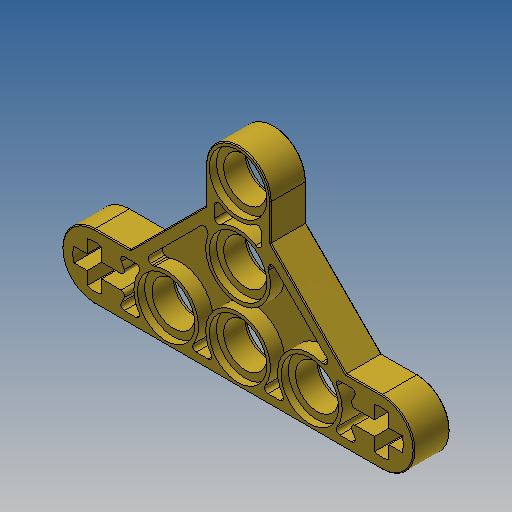
# Autodesk Inventor part: 99773-LtBluishGray
Saved by Autodesk Inventor 2025 (Build 290162010, 162A)
## iProperties
Created: 2014-08-22
Part Number: 99773-LtBluishGray
Material: ABS Plastic
Document SubType Name: Modeling
Designer: D. Kohfeld
Density: 1.06 g/cm^3
Appearance: Yellow
Mass: 0.939287 g
Surface Area: 19.226 cm^2
Volume: 0.88612 cm^3
Author: D. Kohfeld
Autodesk Inventor part; units mm, degrees
ref_plane "YZ Plane" through (0, 0, 0) normal (1, 0, 0) x (0, 1, 0)
ref_plane "XZ Plane" through (0, 0, 0) normal (0, 1, 0) x (-1, 0, 0)
ref_plane "XY Plane" through (0, 0, 0) normal (0, 0, 1) x (1, 0, 0)
sketch "Sketch1" plane through (0, 0, 0) normal (0, 0, 1) x (1, 0, 0)
  circle A0 centre (0, 0) radius 2.4
  circle A1 centre (-8, 0) radius 2.4
  circle A2 centre (-16, 0) radius 2.4 construction
  circle A3 centre (8, 0) radius 2.4
  circle A4 centre (16, 0) radius 2.4 construction
  circle A5 centre (0, 8) radius 2.4
  circle A6 centre (0, 16) radius 2.4
  line L0 (-16, 0) -> (-8, 0) construction
  line L1 (-8, 0) -> (0, 0) construction
  line L2 (0, 0) -> (8, 0) construction
  line L3 (8, 0) -> (16, 0) construction
  line L4 (0, 0) -> (0, 8) construction
  line L5 (0, 8) -> (0, 16) construction
  circle A7 centre (-8, 0) radius 3.6 construction
  circle A8 centre (0, 0) radius 3.6 construction
  circle A9 centre (8, 0) radius 3.6 construction
  circle A10 centre (0, 8) radius 3.6 construction
  circle A11 centre (0, 16) radius 3.6 construction
  line L6 (-3.6, 16) -> (-3.6, 12)
  line L7 (-3.6, 12) -> (-12, 3.6)
  line L8 (-12, 3.6) -> (-16, 3.6)
  arc A12 (-16, 3.6) -> (-16, -3.6) centre (-16, 0) ccw
  line L9 (-16, -3.6) -> (16, -3.6)
  arc A13 (16, -3.6) -> (16, 3.6) centre (16, 0) ccw
  line L10 (16, 3.6) -> (12, 3.6)
  line L11 (12, 3.6) -> (3.6, 12)
  line L12 (3.6, 12) -> (3.6, 16)
  arc A14 (3.6, 16) -> (-3.6, 16) centre (0, 16) ccw
  line L13 (-2.6, 13.51) -> (-2.6, 10.49)
  line L14 (2.6, 13.51) -> (2.6, 10.49)
  arc A15 (2.6, 10.49) -> (-2.6, 10.49) centre (0, 8) ccw
  arc A16 (-2.6, 13.51) -> (2.6, 13.51) centre (0, 16) ccw
  arc A17 (-3.32, 9.3919) -> (3.32, 9.3919) centre (0, 8) ccw
  line L15 (3.32, 9.3919) -> (3.6, 10.4005)
  line L16 (3.6, 10.4005) -> (10.4005, 3.6)
  line L17 (-3.32, 9.3919) -> (-3.6, 10.4005)
  line L18 (-3.6, 10.4005) -> (-10.4005, 3.6)
  arc A18 (2.49, -2.6) -> (-2.49, -2.6) centre (0, 0) ccw
  arc A19 (9.3777, 3.3259) -> (5.51, -2.6) centre (8, 0) ccw
  arc A20 (-5.51, -2.6) -> (-9.3777, 3.3259) centre (-8, 0) ccw
  line L19 (5.51, -2.6) -> (2.49, -2.6)
  line L20 (-2.49, -2.6) -> (-5.51, -2.6)
  line L21 (-10.49, -2.6) -> (-13.51, -2.6)
  line L22 (-10.49, 2.6) -> (-13.51, 2.6)
  arc A21 (-10.49, 2.6) -> (-10.49, -2.6) centre (-8, 0) ccw
  line L23 (-16.8, 2.2627) -> (-16.8, 0.8)
  line L24 (-16.8, 0.8) -> (-18.2627, 0.8)
  line L25 (-18.2627, -0.8) -> (-16.8, -0.8)
  line L26 (-16.8, -0.8) -> (-16.8, -2.2627)
  line L27 (-15.2, -2.2627) -> (-15.2, -0.8)
  line L28 (-15.2, -0.8) -> (-12.49, -0.8)
  line L29 (-15.2, 2.2627) -> (-15.2, 0.8)
  line L30 (-15.2, 0.8) -> (-12.49, 0.8)
  arc A22 (-13.51, -2.6) -> (-13.51, 2.6) centre (-16, 0) ccw
  arc A23 (-15.2, 2.2627) -> (-16.8, 2.2627) centre (-16, 0) ccw
  arc A24 (-18.2627, 0.8) -> (-18.2627, -0.8) centre (-16, 0) ccw
  arc A25 (-16.8, -2.2627) -> (-15.2, -2.2627) centre (-16, 0) ccw
  line L31 (13.51, 2.6) -> (10.49, 2.6)
  line L32 (10.49, -2.6) -> (13.51, -2.6)
  arc A26 (10.49, -2.6) -> (10.49, 2.6) centre (8, 0) ccw
  arc A27 (13.51, 2.6) -> (13.51, -2.6) centre (16, 0) ccw
  line L33 (15.2, 2.2627) -> (15.2, 0.8)
  line L34 (15.2, 0.8) -> (12.49, 0.8)
  line L35 (15.2, -2.2627) -> (15.2, -0.8)
  line L36 (15.2, -0.8) -> (12.49, -0.8)
  line L37 (16.8, -2.2627) -> (16.8, -0.8)
  line L38 (16.8, -0.8) -> (18.2627, -0.8)
  line L39 (18.2627, 0.8) -> (16.8, 0.8)
  line L40 (16.8, 0.8) -> (16.8, 2.2627)
  arc A28 (16.8, 2.2627) -> (15.2, 2.2627) centre (16, 0) ccw
  arc A29 (18.2627, -0.8) -> (18.2627, 0.8) centre (16, 0) ccw
  arc A30 (15.2, -2.2627) -> (16.8, -2.2627) centre (16, 0) ccw
  line L41 (-10.4005, 3.6) -> (-9.3777, 3.3259)
  line L42 (10.4005, 3.6) -> (9.3777, 3.3259)
  dimension "d0" = 8
  dimension "d1" = 4.8
  dimension "d2" = 4.8
  dimension "d3" = 7.2
  dimension "d5" = 1
  dimension "d6" = 1
  dimension "d7" = 1.6
  dimension "d8" = 1.6
  dimension "d17" = 4
  dimension "d18" = 1.131
  dimension "d20" = 15
  constraints: 86 end point, 64 point on circle, 31 centre point, 26 equal radius, 20 equal length, 15 parallel, 12 horizontal alignment, 11 coincident, 9 tangent, 6 collinear, 6 perpendicular, 4 vertical, 3 horizontal, 3 vertical alignment, 2 concentric
  measures "d0" distance of L0.end L1.end
  measures "d1" diameter of A1
  measures "d2" diameter of A2
  measures "d3" diameter of A11
  measures "d5" distance between parallel lines of L6 L13
  measures "d6" distance between parallel lines of L8 L22
  measures "d7" distance between parallel lines of L29 L23
  measures "d8" distance between parallel lines of L40 L33
  measures "d17" vertical distance of L5.end L6.end
  measures "d18" distance between parallel lines of L7 L18
  measures "d20" angle of L8 L41
extrude "Extrusion1" add sketch "Sketch1" along normal mid plane 4
extrude "Extrusion2" add sketch "Sketch1" along normal mid plane 0.8 contours A16 L14 A15 L13 | A17 L15 L16 L42 A19 L19 A18 L20 A20 L41 L18 L17
sketch "Sketch2" plane through (0, 0, 2) normal (0, 0, 1) x (1, 0, 0)
  circle A0 centre (0, 16) radius 2.4 projected
  circle A1 centre (0, 8) radius 2.4 projected
  circle A2 centre (8, 0) radius 2.4 projected
  circle A3 centre (-8, 0) radius 2.4 projected
  circle A4 centre (0, 0) radius 2.4 projected
  arc A5 (10.49, -2.6) -> (10.49, 2.6) centre (8, 0) ccw projected
  arc A6 (-2.6, 13.51) -> (2.6, 13.51) centre (0, 16) ccw projected
  arc A7 (2.6, 10.49) -> (-2.6, 10.49) centre (0, 8) ccw projected
  arc A8 (-10.49, 2.6) -> (-10.49, -2.6) centre (-8, 0) ccw projected
  circle A9 centre (-8, 0) radius 3.2
  circle A10 centre (0, 0) radius 3.2
  circle A11 centre (8, 0) radius 3.2
  circle A12 centre (0, 8) radius 3.2
  circle A13 centre (0, 16) radius 3.2
  dimension "d13" = 6.4
  constraints: 5 centre point, 5 coincident, 4 equal radius
  measures "d13" diameter of A13
extrude "Extrusion3" cut sketch "Sketch2" against normal blind 0.8
mirror "Mirror1" about plane through (0, 0, 0) normal (0, 0, 1) of "Extrusion3"
fillet "Fillet1" radius 0.1 20 edges at (-19.6, 0, 2) (0, -3.6, 2) (19.6, 0, 2) (14, 3.6, 2) (-14, 3.6, 2) (-7.8, 7.8, 2) (0, 19.6, 2) (3.6, 14, 2) (-3.6, 14, 2) (7.8, 7.8, 2) (-19.6, 0, -2) (0, -3.6, -2) (19.6, 0, -2) (14, 3.6, -2) (-14, 3.6, -2) (-7.8, 7.8, -2) (3.6, 14, -2) (-3.6, 14, -2) (0, 19.6, -2) (7.8, 7.8, -2)
fillet "Fillet1" radius 0.4 44 edges at (-12.49, -0.8, 0) (-13.51, -2.6, 0) (-10.49, -2.6, 0) (-13.51, 2.6, 0) (-10.49, 2.6, 0) (-12.49, 0.8, 0) (-9.3777, 3.3259, 1.2) (-5.51, -2.6, 1.2) (-2.49, -2.6, 1.2) (-10.4005, 3.6, 1.2) (-3.6, 10.4005, 1.2) (-3.32, 9.3919, 1.2) (2.6, 10.49, 1.2) (-2.6, 10.49, 1.2) (3.6, 10.4005, 1.2) (3.32, 9.3919, 1.2) (10.4005, 3.6, 1.2) (9.3777, 3.3259, 1.2) (10.49, 2.6, 0) (13.51, 2.6, 0) (12.49, 0.8, 0) (12.49, -0.8, 0) (13.51, -2.6, 0) (10.49, -2.6, 0) (5.51, -2.6, 1.2) (2.49, -2.6, 1.2) (-2.6, 13.51, 1.2) (2.6, 13.51, 1.2) (10.4005, 3.6, -1.2) (9.3777, 3.3259, -1.2) (5.51, -2.6, -1.2) (2.49, -2.6, -1.2) (-2.49, -2.6, -1.2) (-5.51, -2.6, -1.2) (-9.3777, 3.3259, -1.2) (-10.4005, 3.6, -1.2) (-3.6, 10.4005, -1.2) (-3.32, 9.3919, -1.2) (3.6, 10.4005, -1.2) (3.32, 9.3919, -1.2) (2.6, 10.49, -1.2) (2.6, 13.51, -1.2) (-2.6, 13.51, -1.2) (-2.6, 10.49, -1.2)
equation "\"d0\" = lu"
equation "\"d1\" = tpd"
equation "\"d2\" = kd"
equation "\"d3\" = tlad"
equation "\"d6\" = d5"
equation "\"d7\" = axlet"
equation "\"d8\" = axlet"
equation "\"d9\" = 0.5 * lu"
equation "\"d13\" = tsd"
equation "\"d14\" = tsl"
equation "\"d16\" = lf"
equation "\"d21\" = tf"
equation "\"lf\" = 0.1"
equation "\"tf\" = 0.4"
equation "\"lu\" = 8"
equation "\"tpd\" = 4.8"
equation "\"kd\" = 4.8"
equation "\"tlad\" = 7.2"
equation "\"axlet\" = 1.6"
equation "\"tsd\" = 6.4"
equation "\"tsl\" = 0.8"
body "Solid1"
